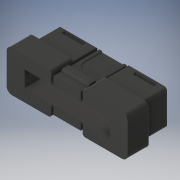
# Autodesk Inventor part: Conector
Saved by Autodesk Inventor 2017 SP1 (Build 210196100, 196)
## iProperties
Created: 2016-11-30
Part Number: Conector
Material: PBT Plastic
Document SubType Name: Modeling
Designer: rbibb
Density: 1.31 g/cm^3
Appearance: Smooth - Black
Author: rbibb
Autodesk Inventor part; units mm, degrees
ref_plane "YZ Plane" through (0, 0, 0) normal (1, 0, 0) x (0, 1, 0)
ref_plane "XZ Plane" through (0, 0, 0) normal (0, 1, 0) x (-1, 0, 0)
ref_plane "XY Plane" through (0, 0, 0) normal (0, 0, 1) x (1, 0, 0)
sketch "Sketch1" plane through (0, 0, 0) normal (0, 0, 1) x (1, 0, 0)
  line L0 (0, 0) -> (0, 8.128)
  line L1 (0, 8.128) -> (-6.604, 8.128)
  line L2 (-6.604, 8.128) -> (-6.604, 4.318)
  line L3 (-6.604, 4.318) -> (-6.604, 4.318)
  line L4 (-7.62, 5.334) -> (-7.62, 8.636)
  line L5 (-8.89, 9.906) -> (-26.67, 9.906)
  line L6 (-29.21, 7.366) -> (-29.21, 0)
  line L7 (-29.21, 0) -> (0, 0)
  arc A0 (-7.62, 5.334) -> (-6.604, 4.318) centre (-6.604, 5.334) ccw
  arc A1 (-7.62, 8.636) -> (-8.89, 9.906) centre (-8.89, 8.636) ccw
  arc A2 (-26.67, 9.906) -> (-29.21, 7.366) centre (-26.67, 7.366) ccw
  dimension "d0" = 29.21
  dimension "d1" = 7.62
  dimension "d2" = 1.016
  dimension "d3" = 5.588
  dimension "d4" = 9.906
  dimension "d5" = 8.128
  dimension "d6" = 1.016
  dimension "d7" = 1.27
  dimension "d8" = 2.54
  constraints: 16 end point, 7 perpendicular, 6 point on circle, 6 tangent, 3 centre point, 1 vertical
  measures "d0" distance between parallel lines of L0 L6
  measures "d1" distance between parallel lines of L0 L4
  measures "d2" distance between parallel lines of L4 L2
  measures "d3" distance between parallel lines of L5 L3
  measures "d4" distance between parallel lines of L5 L7
  measures "d5" distance between parallel lines of L7 L1
  measures "d6" radius of A0
  measures "d7" radius of A1
  measures "d8" radius of A2
extrude "Extrusion1" add sketch "Sketch1" along normal blind 22.225
mirror "Mirror1" about plane through (0, 0, 0) normal (1, 0, 0) of "Extrusion1"
mirror "Mirror2" about plane through (-29.21, 0, 0) normal (0, -1, 0) of "Extrusion1", "Mirror1"
sketch "Sketch2" plane through (0, 0, 22.225) normal (0, 0, 1) x (1, 0, 0)
  line L0 (-20.574, 3.937) -> (20.574, 3.937)
  line L1 (20.574, 3.937) -> (20.574, -3.937)
  line L2 (20.574, -3.937) -> (-20.574, -3.937)
  line L3 (-20.574, -3.937) -> (-20.574, 3.937)
  line L4 (-29.21, 7.366) -> (-29.21, -7.366) projected
  line L5 (29.21, -7.366) -> (29.21, 7.366) projected
  line L6 (-8.89, 9.906) -> (-26.67, 9.906) projected
  point P0 (0, 0)
  dimension "d11" = 8.636
  dimension "d12" = 8.636
  dimension "d13" = 7.874
  dimension "d14" = 5.969
  constraints: 8 end point, 2 parallel, 1 horizontal, 1 perpendicular
  measures "d11" distance between parallel lines of L4 L3
  measures "d12" distance between parallel lines of L5 L1
  measures "d13" distance between parallel lines of L2 L0
  measures "d14" distance between parallel lines of L6 L0
extrude "Extrusion2" cut sketch "Sketch2" against normal blind 8.382
sketch "Sketch3" plane through (0, 0, 0) normal (0, 0, -1) x (-1, 0, 0)
  line L0 (7.62, 5.334) -> (7.62, 8.636) projected
  line L1 (7.62, 8.509) -> (26.0695, 8.509)
  line L2 (26.0695, 8.509) -> (26.0695, -8.509)
  line L3 (26.0695, -8.509) -> (7.62, -8.509)
  line L4 (7.62, -8.509) -> (7.62, 8.509)
  line L5 (7.62, 8.636) -> (0, 21.0607)
  line L6 (0, 21.0607) -> (53.2045, 21.0607)
  line L7 (53.2045, 21.0607) -> (37.8904, -23.4893)
  line L8 (37.8904, -23.4893) -> (1.8924, -20.7049)
  line L9 (1.8924, -20.7049) -> (7.62, -8.509)
  point P0 (0, 0)
  dimension "d17" = 17.018
  dimension "d19" = 18.4495
  constraints: 18 end point, 2 horizontal, 2 parallel, 1 perpendicular, 1 point on line
  measures "d17" distance of L1.end L2.end
  measures "d19" distance between parallel lines of L2 L4
extrude "Extrusion3" cut sketch "Sketch3" against normal blind 11.938 contours L0 L5 L6 L7 L8 L9 L3 L2 L1
fillet "Fillet1" radius 1.27 2 edges at (-26.0695, 8.509, 5.969) (-26.0695, -8.509, 5.969)
sketch "Sketch4" plane through (0, 0, 0) normal (0, 0, -1) x (-1, 0, 0)
  line L0 (9.5595, 6.223) -> (21.4975, 6.223)
  line L1 (21.4975, 6.223) -> (21.4975, -5.969)
  line L2 (21.4975, -5.969) -> (9.5595, -5.969)
  line L3 (9.5595, -5.969) -> (9.5595, 6.223)
  line L4 (26.0695, -7.239) -> (26.0695, 7.239) projected
  line L5 (7.62, -8.509) -> (24.7995, -8.509) projected
  point P0 (0, 0)
  dimension "d23" = 11.938
  dimension "d24" = 12.192
  dimension "d25" = 4.572
  dimension "d26" = 2.54
  constraints: 8 end point, 2 parallel, 1 horizontal, 1 perpendicular
  measures "d23" distance of L1.end L2.end
  measures "d24" distance of L0.end L1.end
  measures "d25" distance between parallel lines of L4 L1
  measures "d26" distance between parallel lines of L5 L2
extrude "Extrusion4" cut sketch "Sketch4" against normal blind 11.938
ref_plane "Work Plane1" through (0, -7.366, 22.225) normal (-1, 0, 0) x (0, 0, 1)
sketch "Sketch5" plane through (-7.62, 8.509, 11.938) normal (0, 1, 0) x (1, 0, 0)
  line L0 (-4.572, 9.398) -> (-14.732, 9.398)
  line L1 (-14.732, 9.398) -> (-14.732, 10.922)
  line L2 (-14.732, 10.922) -> (-4.572, 10.922)
  line L3 (-4.572, 10.922) -> (-4.572, 9.398)
  line L4 (0, 11.938) -> (0, 0) projected
  line L5 (-1.9395, 11.938) -> (-13.8775, 11.938) projected
  point P0 (7.62, 11.938)
  dimension "d29" = 10.16
  dimension "d30" = 1.524
  dimension "d31" = 4.572
  dimension "d32" = 1.016
  constraints: 8 end point, 2 parallel, 1 horizontal, 1 perpendicular
  measures "d29" distance of L0.start L0.end
  measures "d30" distance of L0.end L1.end
  measures "d31" distance between parallel lines of L4 L3
  measures "d32" distance between parallel lines of L5 L2
extrude "Extrusion5" cut sketch "Sketch5" against normal blind 1.27
mirror "Mirror3" about plane through (0, -7.366, 22.225) normal (-1, 0, 0) of "Extrusion4", "Extrusion3", "Fillet1"
mirror "Mirror4" about plane through (0, -7.366, 22.225) normal (-1, 0, 0) of "Extrusion5"
sketch "Sketch6" plane through (0, 0, 0) normal (0, 0, -1) x (-1, 0, 0)
  line L0 (-6.604, -8.128) -> (-6.604, -4.318) projected
  line L1 (6.604, -7.366) -> (-6.604, -7.366)
  line L2 (-6.604, -7.366) -> (6.604, -7.366)
  line L3 (6.604, -7.366) -> (6.604, -4.318)
  line L4 (6.604, -4.318) -> (-6.604, -4.318)
  line L5 (-6.604, -4.318) -> (-6.604, -7.366)
  point P0 (0, 0)
  constraints: 10 end point, 2 parallel, 1 horizontal, 1 perpendicular
extrude "Extrusion6" cut sketch "Sketch6" against normal blind 13.97
ref_plane "Work Plane2" through (-6.604, 0, 22.225) normal (0, 1, 0) x (1, 0, 0)
mirror "Mirror5" about plane through (-6.604, 0, 22.225) normal (0, 1, 0) of "Extrusion6"
sketch "Sketch7" plane through (-6.604, 8.128, 22.225) normal (0, 1, 0) x (1, 0, 0)
  arc A0 (1.2192, 13.9502) -> (11.9888, 13.9502) centre (6.604, 13.9502) ccw
  line L0 (11.9888, 13.9502) -> (11.9888, 22.225)
  line L1 (1.2192, 13.9502) -> (1.2192, 22.225)
  point P0 (6.604, 22.225)
  constraints: 4 end point, 2 point on circle, 2 vertical, 1 centre point, 1 tangent
extrude "Extrusion7" cut sketch "Sketch7" against normal blind 0.635 fills toward (1.2692, 18.0876) open curves L1 A0 L0
fillet "Fillet2" radius 0.508 3 edges at (-5.3848, 7.493, 4.1374) (5.3848, 7.493, 4.1374) (0, 7.493, 13.6596)
sketch "Sketch8" plane through (-6.604, 7.493, 22.225) normal (0, 1, 0) x (1, 0, 0)
  line L0 (1.7272, 13.9502) -> (1.7272, 22.225) projected
  line L1 (11.4138, 19.7647) -> (1.7272, 19.7647)
  line L2 (1.7272, 19.7647) -> (1.7272, 19.1565)
  line L3 (1.7272, 19.1565) -> (11.4138, 19.1565)
  line L4 (11.4138, 19.1565) -> (11.4138, 19.7647)
  line L5 (2.347, 16.337) -> (11.0268, 16.337)
  line L6 (11.0268, 16.337) -> (11.0268, 15.7288)
  line L7 (11.0268, 15.7288) -> (2.347, 15.7288)
  line L8 (2.347, 15.7288) -> (2.347, 16.337)
  line L9 (10.0317, 12.6328) -> (3.3974, 12.6328)
  line L10 (3.3974, 12.6328) -> (3.3974, 11.7483)
  line L11 (3.3974, 11.7483) -> (10.0317, 11.7483)
  line L12 (10.0317, 11.7483) -> (10.0317, 12.6328)
  point P0 (6.604, 22.225)
  constraints: 24 end point, 6 parallel, 3 horizontal, 3 perpendicular, 1 point on line
extrude "Extrusion8" add sketch "Sketch8" along normal blind 0.2286
chamfer "Chamfer1" distance 0.1778 angle 45 6 edges at (0.1106, 7.7216, 10.4767) (0.1106, 7.7216, 9.5922) (0.0829, 7.7216, 6.4962) (0.0829, 7.7216, 5.888) (-0.0335, 7.7216, 2.4603) (-0.0335, 7.7216, 3.0685)
mirror "Mirror6" about plane through (-6.604, 0, 22.225) normal (0, 1, 0) of "Mirror5", "Extrusion6", "Extrusion7", "Fillet2", "Extrusion8", "Chamfer1"
sketch "Sketch9" plane through (-6.604, 8.128, 22.225) normal (0, 1, 0) x (1, 0, 0)
  line L0 (0, 0) -> (-1.016, 0) projected
  line L1 (13.208, 22.225) -> (13.208, 0) projected
  line L2 (0, 0) -> (13.208, 0)
  line L3 (13.208, 0) -> (13.208, 3.7319)
  line L4 (13.208, 3.7319) -> (0, 3.7319)
  line L5 (0, 3.7319) -> (0, 0)
  line L6 (0, 8.255) -> (0, 0) projected
  line L7 (13.208, 3.7319) -> (0, 3.7319)
  line L8 (0, 3.7319) -> (0, 7.3807)
  line L9 (0, 7.3807) -> (13.208, 7.3807)
  line L10 (13.208, 7.3807) -> (13.208, 3.7319)
  point P0 (6.604, 22.225)
  constraints: 16 end point, 4 parallel, 2 horizontal, 2 perpendicular, 2 point on line
extrude "Extrusion9" add sketch "Sketch9" along normal blind 1.016 contours L1 L4 L6 L9
chamfer "Chamfer2" distance 0.762 angle 45 1 edges at (0, 9.144, 18.4931)
fillet "Fillet3" radius 0.508 6 edges at (0, 9.144, 17.7311) (-25.6975, -8.137, 0) (-26.0695, 0, 0) (-25.6975, 8.137, 0) (-16.2098, 8.509, 0) (-16.2098, -8.509, 0)
ref_plane "Work Plane3" through (-6.604, 0, 22.225) normal (0, 1, 0) x (1, 0, 0)
mirror "Mirror7" about plane through (-6.604, 0, 22.225) normal (0, 1, 0) of "Extrusion9"
body "Solid1"
